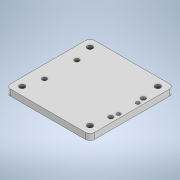
# Autodesk Inventor part: bottom
Saved by Autodesk Inventor 2020 (Build 240168000, 168)
## iProperties
Created: 2022-08-25
Part Number: bottom
Material: Типовые
Document SubType Name: Modeling
Designer: zigma
Density: 1 g/cm^3
Appearance: По умолчанию
Author: zigma
Autodesk Inventor part; units mm, degrees
ref_plane "YZ Plane" through (0, 0, 0) normal (1, 0, 0) x (0, 1, 0)
ref_plane "XZ Plane" through (0, 0, 0) normal (0, 1, 0) x (-1, 0, 0)
ref_plane "XY Plane" through (0, 0, 0) normal (0, 0, 1) x (1, 0, 0)
sketch "Эскиз1" plane through (0, 0, 0) normal (0, 1, 0) x (-1, 0, 0)
  line L0 (0, 0) -> (54.5, 0)
  line L1 (54.5, 0) -> (54.5, -54.5)
  line L2 (54.5, -54.5) -> (0, -54.5)
  line L3 (0, -54.5) -> (0, 0)
  dimension "d0" = 54.5
  dimension "d1" = 54.5
  constraints: 8 end point, 2 parallel, 1 horizontal, 1 perpendicular
  measures "d0" distance of L1.end L2.end
  measures "d1" distance of L0.end L1.end
extrude "Выдавливание1" add sketch "Эскиз1" along normal blind 4
fillet "Сопряжение1" radius 3 4 edges at (0, 2, 0) (0, 2, -54.5) (-54.5, 2, -54.5) (-54.5, 2, 0)
sketch "Эскиз2" plane through (0, 0, 0) normal (0, -1, 0) x (1, 0, 0)
  arc A0 (-54.5, -51.5) -> (-51.5, -54.5) centre (-51.5, -51.5) ccw projected
  line L0 (-54.5, -51.5) -> (-54.5, -3) projected
  line L1 (-54.5, -27.25) -> (0, -27.25) construction
  line L2 (0, -3) -> (0, -51.5) projected
  line L3 (-3, -54.5) -> (-51.5, -54.5) projected
  line L4 (-27.25, -54.5) -> (-27.25, 0) construction
  line L5 (-51.5, 0) -> (-3, 0) projected
  line L6 (-54.5, -51.5) -> (-54.5, -3) projected
  circle A1 centre (-49.25, -49.25) radius 3
  circle A2 centre (-49.25, -5.25) radius 3
  circle A3 centre (-5.25, -49.25) radius 3
  circle A4 centre (-5.25, -5.25) radius 3
  point P0 (0, 0)
  dimension "d13" = 6
  dimension "d34" = 44
  dimension "d35" = 44
  constraints: 4 centre point, 4 end point, 4 midpoint, 3 symmetric about line, 2 other
  measures "d13" diameter of A1
  measures "d34" distance of A2.centre A1.centre
  measures "d35" distance of A3.centre A1.centre
extrude "Выдавливание2" cut sketch "Эскиз2" against normal blind 2
sketch "Эскиз3" plane through (0, 2, 0) normal (0, -1, 0) x (1, 0, 0)
  circle A0 centre (-49.25, -49.25) radius 1.75
  line L0 (-54.5, -51.5) -> (-54.5, -3) projected
  line L1 (-54.5, -27.25) -> (0, -27.25) construction
  line L2 (0, -3) -> (0, -51.5) projected
  line L3 (-3, -54.5) -> (-51.5, -54.5) projected
  line L4 (-27.25, -54.5) -> (-27.25, 0) construction
  line L5 (-51.5, 0) -> (-3, 0) projected
  circle A1 centre (-49.25, -5.25) radius 1.75
  circle A2 centre (-5.25, -49.25) radius 1.75
  circle A3 centre (-5.25, -5.25) radius 1.75
  circle A4 centre (-49.25, -49.25) radius 3 construction
  circle A5 centre (-49.25, -49.25) radius 3
  point P0 (0, 0)
  point P1 (-45.0293, -48.6853)
  point P2 (-51.4707, -47.8147)
  dimension "d9" = 3.5
  constraints: 5 centre point, 4 end point, 4 midpoint, 3 symmetric about line, 2 coincident, 3 other
  measures "d9" diameter of A0
extrude "Выдавливание3" cut sketch "Эскиз3" against normal blind 2 contours A0 | A1 | A2 | A3
sketch "Эскиз4" plane through (0, 4, 0) normal (0, 1, 0) x (1, 0, 0)
  line L0 (-54.5, 51.5) -> (-54.5, 3) projected
  line L1 (0, 3) -> (0, 51.5) construction
  line L2 (-51.5, 0) -> (-3, 0) projected
  line L3 (-3, 54.5) -> (-51.5, 54.5) projected
  line L4 (-49.5, 14.5) -> (0, 14.5) construction
  line L5 (0, 14.5) -> (0, 40) construction
  line L6 (0, 40) -> (-49.5, 40) construction
  line L7 (-49.5, 40) -> (-49.5, 14.5) construction
  line L8 (-46.25, 16.75) -> (-3.25, 16.75) construction
  line L9 (-3.25, 16.75) -> (-3.25, 37.75) construction
  line L10 (-3.25, 37.75) -> (-46.25, 37.75) construction
  line L11 (-46.25, 37.75) -> (-46.25, 16.75) construction
  line L12 (-24.75, 14.5) -> (-24.75, 40) construction
  line L13 (0, 27.25) -> (-24.75, 27.25) construction
  line L14 (-24.75, 16.75) -> (-24.75, 37.75) construction
  line L15 (-3.25, 27.25) -> (-24.75, 27.25) construction
  circle A0 centre (-46.25, 16.75) radius 1.5
  circle A1 centre (-46.25, 37.75) radius 1.5
  circle A2 centre (-3.25, 37.75) radius 1.5
  circle A3 centre (-3.25, 16.75) radius 1.5
  line L16 (-27.25, 27.25) -> (-21.7344, 27.25) construction
  point P0 (0, 0)
  dimension "d17" = 49.5
  dimension "d18" = 25.5
  dimension "d19" = 43
  dimension "d20" = 21
  dimension "d21" = 3
  dimension "d22" = 3
  dimension "d23" = 3
  dimension "d24" = 3
  dimension "d36" = 2.25
  dimension "d37" = 3.25
  dimension "d40" = 3.25
  dimension "d41" = 2.25
  dimension "d42" = 2.25
  dimension "d43" = 3.25
  dimension "d44" = 3.25
  dimension "d45" = 2.25
  constraints: 26 end point, 9 midpoint, 4 centre point, 4 parallel, 3 horizontal, 2 perpendicular, 1 coincident
  measures "d17" distance of L6.end L5.end
  measures "d18" distance of L5.end L4.end
  measures "d19" distance of L10.end L9.end
  measures "d20" distance of L9.end L8.end
  measures "d21" diameter of A0
  measures "d22" diameter of A1
  measures "d23" diameter of A2
  measures "d24" diameter of A3
  measures "d36" distance from line of L4 A3.centre
  measures "d37" distance from line of L5 A3.centre
  measures "d40" distance from line of L5 A2.centre
  measures "d41" distance from line of L6 A2.centre
  measures "d42" distance from line of L4 A0.centre
  measures "d43" distance from line of L7 A0.centre
  measures "d44" distance from line of L7 A1.centre
  measures "d45" distance from line of L6 A1.centre
extrude "Выдавливание4" cut sketch "Эскиз4" against normal blind 4
sketch "Эскиз5" plane through (0, 0, 0) normal (0, -1, 0) x (1, 0, 0)
  circle A0 centre (-3.25, -16.75) radius 1.5 projected
  circle A1 centre (-3.25, -16.75) radius 2.25 construction
  line L0 (-1, -16.75) -> (-2.125, -18.6986)
  line L1 (-2.125, -18.6986) -> (-4.375, -18.6986)
  line L2 (-4.375, -18.6986) -> (-5.5, -16.75)
  line L3 (-5.5, -16.75) -> (-4.375, -14.8014)
  line L4 (-4.375, -14.8014) -> (-2.125, -14.8014)
  line L5 (-2.125, -14.8014) -> (-1, -16.75)
  circle A2 centre (-3.25, -37.75) radius 1.5 projected
  circle A3 centre (-3.25, -37.75) radius 1.5
  circle A4 centre (-46.25, -37.75) radius 1.5 projected
  circle A5 centre (-46.25, -37.75) radius 1.5
  circle A6 centre (-46.25, -16.75) radius 1.5 projected
  circle A7 centre (-46.25, -16.75) radius 1.5
  line L6 (-1, -37.75) -> (-2.125, -39.6986)
  line L7 (-2.125, -39.6986) -> (-4.375, -39.6986)
  line L8 (-4.375, -39.6986) -> (-5.5, -37.75)
  line L9 (-5.5, -37.75) -> (-4.375, -35.8014)
  line L10 (-4.375, -35.8014) -> (-2.125, -35.8014)
  line L11 (-2.125, -35.8014) -> (-1, -37.75)
  line L12 (-44, -37.75) -> (-45.125, -39.6986)
  line L13 (-45.125, -39.6986) -> (-47.375, -39.6986)
  line L14 (-47.375, -39.6986) -> (-48.5, -37.75)
  line L15 (-48.5, -37.75) -> (-47.375, -35.8014)
  line L16 (-47.375, -35.8014) -> (-45.125, -35.8014)
  line L17 (-45.125, -35.8014) -> (-44, -37.75)
  line L18 (-44, -16.75) -> (-45.125, -18.6986)
  line L19 (-45.125, -18.6986) -> (-47.375, -18.6986)
  line L20 (-47.375, -18.6986) -> (-48.5, -16.75)
  line L21 (-48.5, -16.75) -> (-47.375, -14.8014)
  line L22 (-47.375, -14.8014) -> (-45.125, -14.8014)
  line L23 (-45.125, -14.8014) -> (-44, -16.75)
  line L24 (-44, -16.75) -> (-48.5, -16.75) construction
  line L25 (-44, -37.75) -> (-48.5, -37.75) construction
  line L26 (-1, -37.75) -> (-5.5, -37.75) construction
  line L27 (-1, -16.75) -> (-5.5, -16.75) construction
  point P0 (0, 0)
  dimension "d27" = 4.5
  constraints: 56 end point, 8 coincident, 4 horizontal, 3 centre point, 3 midpoint, 1 horizontal alignment, 15 other
extrude "Выдавливание5" cut sketch "Эскиз5" against normal blind 2 contours A0 | L0 L1 L2 L3 L4 L5 | A2 | A4 | A6 | L6 L7 L8 L9 L10 L11 | L12 L13 L14 L15 L16 L17 | L18 L19 L20 L21 L22 L23
sketch "Эскиз6" plane through (0, 0, 0) normal (0, -1, 0) x (1, 0, 0)
  circle A0 centre (-2.5, -33.5) radius 1.25
  line L0 (-2.5, -33.5) -> (-2.5, -21) construction
  circle A1 centre (-2.5, -21) radius 1.25
  line L1 (0, -3) -> (0, -51.5) projected
  line L2 (0, -3) -> (0, -51.5) projected
  line L3 (0, -27.25) -> (-19.5358, -27.25) construction
  point P0 (0, 0)
  point P1 (-2.5, -27.25)
  dimension "d46" = 2.5
  dimension "d47" = 12.5
  dimension "d48" = 2.5
  dimension "d49" = 2.5
  constraints: 4 end point, 2 centre point, 2 midpoint, 1 coincident, 1 horizontal, 1 point on line, 1 vertical
  measures "d46" diameter of A0
  measures "d47" distance of L0.start L0.end
  measures "d48" diameter of A1
  measures "d49" distance between parallel lines of L1 L0
extrude "Выдавливание6" cut sketch "Эскиз6" against normal blind 4
equation "\"d0\" = d1"
equation "\"d22\" = d21"
equation "\"d23\" = d21"
equation "\"d24\" = d21"
equation "\"d36\" = d42"
equation "\"d37\" = d43"
equation "\"d40\" = d43"
equation "\"d41\" = d42"
equation "\"d44\" = d43"
equation "\"d45\" = d42"
